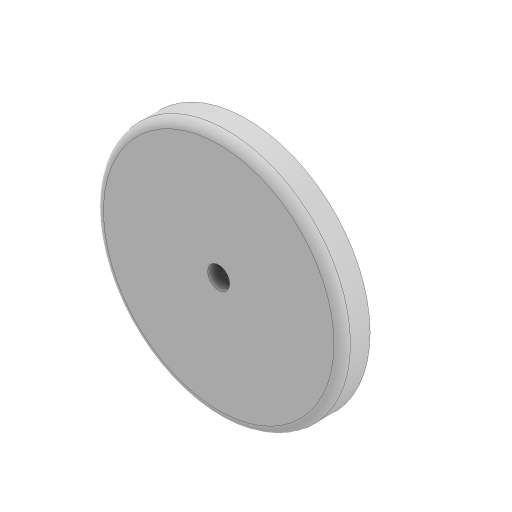
# Autodesk Inventor part: wheel_mrrover
Saved by Autodesk Inventor 2024 (Build 280153000, 153)
## iProperties
Created: 2023-09-15
Part Number: wheel_mrrover
Material: Generic
Document SubType Name: Modeling
Designer: chris
Density: 1 g/cm^3
Appearance: Default
Author: chris
Autodesk Inventor part; units mm, degrees
ref_plane "YZ Plane" through (0, 0, 0) normal (1, 0, 0) x (0, 1, 0)
ref_plane "XZ Plane" through (0, 0, 0) normal (0, 1, 0) x (-1, 0, 0)
ref_plane "XY Plane" through (0, 0, 0) normal (0, 0, 1) x (1, 0, 0)
sketch "Sketch1" plane through (0, 0, 0) normal (0, 0, 1) x (1, 0, 0)
  circle A0 centre (0, 0) radius 3.925
  circle A1 centre (0, 0) radius 2
  dimension "d0" = 7.85
  dimension "d1" = 4
  constraints: 2 centre point, 2 coincident
  measures "d0" diameter of A0
  measures "d1" diameter of A1
extrude "Extrusion1" add sketch "Sketch1" along normal blind 7
sketch "Sketch2" plane through (0, 0, 7) normal (0, 0, 1) x (1, 0, 0)
  circle A0 centre (0, 0) radius 22.5
  circle A1 centre (0, 0) radius 2 projected
  dimension "d4" = 45
  constraints: 1 centre point, 1 coincident
  measures "d4" diameter of A0
extrude "Extrusion2" add sketch "Sketch2" along normal blind 5.08
fillet "Fillet1" radius 1.5 1 edges at (-22.5, 0, 12.08)
sketch "Sketch4" plane through (0, 0, 7) normal (0, 0, -1) x (-1, 0, 0)
  circle A0 centre (0, 0) radius 3.925
  circle A1 centre (0, 0) radius 6.35
  dimension "d10" = 12.7
  constraints: 2 centre point, 2 coincident
  measures "d10" diameter of A1
extrude "Extrusion4" add sketch "Sketch4" along normal blind 1.5
sketch "Sketch5" plane through (0, 0, 0) normal (0, 0, -1) x (-1, 0, 0)
  circle A0 centre (0, 0) radius 3.925 projected
  circle A1 centre (0, 0) radius 2 projected
fillet "Fillet2" radius 1 1 edges at (6.35, 0, 5.5)
extrude "Extrusion5" add sketch "Sketch5" along normal blind 1.5
body "Solid1"
